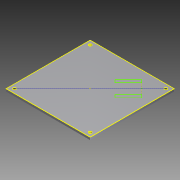
# Autodesk Inventor part: Bottom_Platform
Saved by Autodesk Inventor 2012 (Build 160160000, 160)
## iProperties
Created: 2012-10-03
Part Number: Bottom_Platform
Material: Default
Document SubType Name: Modeling
Designer: agmlego
Density: 1 g/cm^3
Author: agmlego
Autodesk Inventor part; units mm, degrees
ref_plane "YZ Plane" through (0, 0, 0) normal (1, 0, 0) x (0, 1, 0)
ref_plane "XZ Plane" through (0, 0, 0) normal (0, 1, 0) x (-1, 0, 0)
ref_plane "XY Plane" through (0, 0, 0) normal (0, 0, 1) x (1, 0, 0)
sketch "Sketch1" plane through (0, 0, 0) normal (0, 0, 1) x (1, 0, 0)
  line L0 (-50, 50) -> (50, 50)
  line L1 (50, 50) -> (50, -50)
  line L2 (50, -50) -> (-50, -50)
  line L3 (-50, -50) -> (-50, 50)
  point P0 (0, 0)
  dimension "d0" = 100
  dimension "d1" = 50
  dimension "d2" = 50
  constraints: 8 end point, 2 parallel, 2 perpendicular, 1 horizontal
  measures "d0" distance of L2.end L0.start
  measures "d1" distance from line of L0 point (0, 0)
  measures "d2" distance from line of point (0, 0) L3
extrude "Extrusion1" add sketch "Sketch1" along normal blind 3
hole "Hole1" at (-45, 45, 3) direction (0, 0, -1) diameter 3.4 end through all clearance for "Flat Head Machine Screw" size "M3" standard "Ansi Metric M Profile"
hole "Hole2" at (45, 45, 3) direction (0, 0, -1) diameter 3.4 end through all clearance for "Flat Head Machine Screw" size "M3" standard "Ansi Metric M Profile"
hole "Hole3" at (45, -45, 3) direction (0, 0, -1) diameter 3.4 end through all clearance for "Flat Head Machine Screw" size "M3" standard "Ansi Metric M Profile"
hole "Hole4" at (-45, -45, 3) direction (0, 0, -1) diameter 3.4 end through all clearance for "Flat Head Machine Screw" size "M3" standard "Ansi Metric M Profile"
sketch "Sketch2" plane through (0, 0, 3) normal (0, 0, 1) x (1, 0, 0)
  circle A0 centre (-45, -45) radius 1.7 projected
  circle A1 centre (45, -45) radius 1.7 projected
  circle A2 centre (45, 45) radius 1.7 projected
  circle A3 centre (-45, 45) radius 1.7 projected
  line L0 (50, 50) -> (50, -50) projected
  line L1 (-50, 50) -> (50, 50) projected
  line L2 (-50, -50) -> (-50, 50) projected
  line L3 (50, -50) -> (-50, -50) projected
  line L4 (21.5055, 39.8463) -> (5.6322, 23.9731)
  line L5 (5.6322, 23.9731) -> (8.6635, 20.9418)
  line L6 (8.6635, 20.9418) -> (24.5367, 36.8151)
  line L7 (24.5367, 36.8151) -> (21.5055, 39.8463)
  line L8 (36.8151, 24.5367) -> (20.9418, 8.6635)
  line L9 (20.9418, 8.6635) -> (23.9731, 5.6322)
  line L10 (23.9731, 5.6322) -> (39.8463, 21.5055)
  line L11 (39.8463, 21.5055) -> (36.8151, 24.5367)
  line L12 (45, 45) -> (-45, -45) construction
  line L13 (24.5367, 36.8151) -> (36.8151, 24.5367) construction
  point P0 (0, 0)
  point P1 (30.6759, 30.6759)
  constraints: 20 end point, 4 equal length, 3 collinear, 3 parallel, 3 perpendicular, 2 point on line, 1 midpoint
equation "\"d1\" = 0.5 * d0"
equation "\"d2\" = d1"
body "Solid1"
